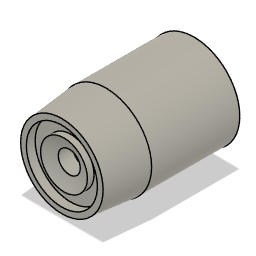
_idler cup.9769f4ec-4f81-49af-b51b-54e774b655a3 (Autodesk Fusion 360 design; units mm, degrees)
Autodesk Fusion 360 part; units mm, degrees
sketch "Sketch1" plane through (0, 0, 0) normal (0, 0, 1) x (1, 0, 0)
  circle A0 centre (0, 0) radius 5.3
  circle A1 centre (0, 0) radius 8.05
  circle A2 centre (0, 0) radius 10.35
  circle A3 centre (0, 0) radius 2.5
  circle A4 centre (0, 0) radius 3
  dimension "d1" = 10.6
  dimension "d2" = 16.1
  dimension "d3" = 20.7
  dimension "d8" = 5
  dimension "d9" = 6
  constraint coincident A0.centre A1.centre
  constraint concentric A0 A1
  constraint concentric A0 A2
  constraint concentric A1 A3
  constraint concentric A0 A4
  measures "d1" diameter of A0
  measures "d2" diameter of A1
  measures "d3" diameter of A2
  measures "d8" diameter of A3
  measures "d9" diameter of A4
extrude "Extrude1" add sketch "Sketch1" along normal blind 30 contours A0 | A2 | A4 makes body 1 at (10.2986, -1.0305, 20) makes body 2 at (5.2737, -0.5277, 20)
extrude "Extrude2" add sketch "Sketch1" along normal blind 28 contours A1 bodies 1 2
extrude "Extrude3" cut sketch "Sketch1" along normal blind 25 contours A3 | A4 bodies 1
chamfer "Chamfer1" distance 1 distance2 10 1 edges at (-9.6496, -3.7427, 30) measured on face at (9.5148, -0.9141, 30) on bodies 1
sketch "Sketch2" plane through (0, 0, 0) normal (1, 0, 0) x (0, 0, -1)
  arc A0 (-38, -10) -> (-28, 0) centre (-38, 0) ccw
  line L0 (-28, 0) -> (-38, 0)
  line L1 (-38, 0) -> (-38, -10)
  line L2 (-1.75, 0) -> (-22.5, 0)
  dimension "d14" = 10
  dimension "d15" = 38
  constraint coincident A0.centre L0.end
  constraint horizontal L0
  constraint perpendicular L0 L1
  constraint coincident A0.centre L2
  measures "d14" radius of A0
  measures "d15" distance of A0.centre origin
revolve "Revolve1" cut sketch "Sketch2" angle 360 about axis through (0, 0, 28) along (0, 0, 1) bodies 1
equation "d8 = draadstang - 2 * draadstangtolerance"
equation "d9 = draadstang"
equation "draadstang = 6 mm"
equation "draadstangtolerance = 0.5 mm"
